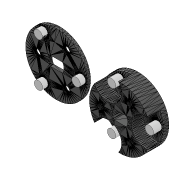
# Autodesk Inventor part: 3
Saved by Autodesk Inventor 2022 (Build 260153000, 153)
## iProperties
Created: 2022-11-30
Part Number: 3
Material: Generisch
Document SubType Name: Modeling
Designer: diederichbenedict
Density: 1 g/cm^3
Appearance: Vorgabe
Author: diederichbenedict
Autodesk Inventor part; units mm, degrees
ref_plane "YZ Plane" through (0, 0, 0) normal (1, 0, 0) x (0, 1, 0)
ref_plane "XZ Plane" through (0, 0, 0) normal (0, 1, 0) x (-1, 0, 0)
ref_plane "XY Plane" through (0, 0, 0) normal (0, 0, 1) x (1, 0, 0)
sketch "Skizze1" plane through (79.33, -93.671, 1.997) normal (0, 0, 1) x (1, 0, 0)
  circle A0 centre (3.4237, 11.9039) radius 1.273 projected
  circle A1 centre (16.9127, 4.1271) radius 1.2955 projected
  circle A2 centre (3.4059, -3.6937) radius 1.3406 projected
  circle A3 centre (3.4237, 11.9039) radius 1.5
  circle A4 centre (16.9127, 4.1271) radius 1.5
  circle A5 centre (3.4059, -3.6937) radius 1.5
  point P0 (-79.33, 93.671)
  dimension "d0" = 3
  dimension "d1" = 3
  dimension "d2" = 3
  constraints: 3 centre point
  measures "d0" diameter of A3
  measures "d1" diameter of A4
  measures "d2" diameter of A5
extrude "Extrusion1" add sketch "Skizze1" along normal blind 3 contours A0 | A1 | A2 | A3 | A4 | A5
sketch "Skizze2" plane through (65.788, -88.308, 1.198) normal (0, 0, 1) x (1, 0, 0)
  circle A0 centre (-11.1016, 6.6961) radius 1.4233 projected
  circle A1 centre (-10.9854, -8.9781) radius 1.2319 projected
  circle A2 centre (2.4601, -1.2) radius 1.287 projected
  circle A3 centre (-11.1016, 6.6961) radius 1.5
  circle A4 centre (2.4601, -1.2) radius 1.5
  circle A5 centre (-10.9854, -8.9781) radius 1.5
  point P0 (-65.788, 88.308)
  dimension "d5" = 3
  dimension "d6" = 3
  dimension "d7" = 3
  constraints: 3 centre point
  measures "d5" diameter of A3
  measures "d6" diameter of A4
  measures "d7" diameter of A5
extrude "Extrusion2" add sketch "Skizze2" along normal blind 2 contours A0 | A1 | A2 | A3 | A4 | A5
